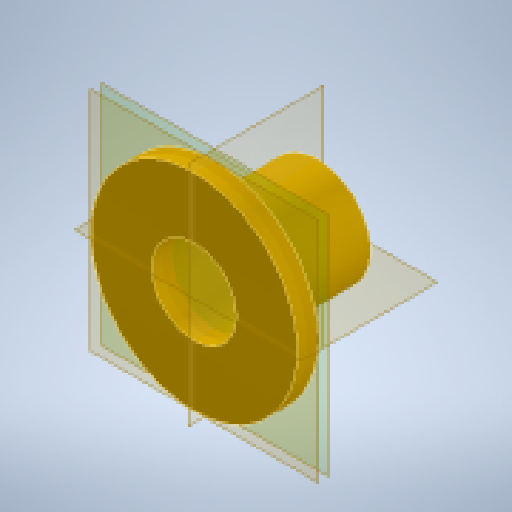
# Autodesk Inventor part: porca_roscada_trapezoidal_001
Saved by Autodesk Inventor 2026 (Build 300175000, 175)
## iProperties
Created: 2025-11-26
Part Number: porca_roscada_trapezoidal_001
Material: Aluminum 6061
Document SubType Name: Modeling
Designer: Carlos Dias
Density: 2.7 g/cm^3
Appearance: Gold
Author: Carlos Dias
Autodesk Inventor part; units mm, degrees
sketch "Sketch1" plane through (0, 0, 0) normal (0, 0, 1) x (1, 0, 0)
  circle A0 centre (0, 0) radius 4.1
  circle A1 centre (0, 0) radius 10
  dimension "d0" = 8.2
  dimension "d7" = 20
  constraints: 2 centre point, 2 coincident
  measures "d0" diameter of A0
  measures "d7" diameter of A1
extrude "Extrusion7" add sketch "Sketch1" along normal mid plane 2
sketch "Sketch5" plane through (0, 0, -1) normal (0, 0, -1) x (-1, 0, 0)
  circle A0 centre (0, 0) radius 4.1 projected
  circle A1 centre (0, 0) radius 4.6
  dimension "d30" = 0.5
  constraints: 1 centre point
  measures "d30" radial gap between concentric circles of A0 A1
extrude "Extrusion8" add sketch "Sketch5" along normal blind 10
body "Solid3"
